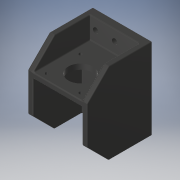
# Autodesk Inventor part: nema17_holder_z
Saved by Autodesk Inventor 2018 (Build 220112000, 112)
## iProperties
Created: 2018-06-01
Part Number: nema17_holder_z
Material: Plastic, Opaque Black
Document SubType Name: Modeling
Designer: Z. Deniz
Density: 0.952 g/cm^3
Appearance: Smooth - Black
Author: Z. Deniz
Autodesk Inventor part; units mm, degrees
ref_plane "YZ Plane" through (0, 0, 0) normal (1, 0, 0) x (0, 1, 0)
ref_plane "XZ Plane" through (0, 0, 0) normal (0, 1, 0) x (-1, 0, 0)
ref_plane "XY Plane" through (0, 0, 0) normal (0, 0, 1) x (1, 0, 0)
sketch "Sketch1" plane through (0, 0, 0) normal (0, 0, 1) x (1, 0, 0)
  line L0 (0, 0) -> (45, 0)
  line L1 (45, 0) -> (45, 75)
  line L2 (45, 75) -> (0, 75)
  line L3 (0, 75) -> (0, 0)
  line L4 (0, 55) -> (45, 55)
  line L5 (0, 50) -> (45, 50)
  line L6 (0, 75) -> (-5, 75)
  line L7 (-5, 75) -> (-5, 0)
  line L8 (-5, 0) -> (0, 0)
  line L9 (45, 75) -> (50, 75)
  line L10 (50, 75) -> (50, 0)
  line L11 (50, 0) -> (45, 0)
  dimension "d0" = 45
  dimension "d1" = 75
  dimension "d2" = 20
  dimension "d3" = 5
  dimension "d4" = 5
  dimension "d5" = 5
  constraints: 24 end point, 7 point on line, 6 perpendicular, 3 parallel, 1 horizontal
  measures "d0" distance of L2.end L1.end
  measures "d1" distance of L1.end L0.end
  measures "d2" distance between parallel lines of L4 L2
  measures "d3" distance between parallel lines of L5 L4
  measures "d4" distance of L2.end L6.end
  measures "d5" distance of L1.end L9.end
extrude "Extrusion1" add sketch "Sketch1" along normal blind 15 contours L3 L5 L1 L0 | L3 L2 L1 L4
extrude "Extrusion2" add sketch "Sketch1" along normal blind 60 contours L8 L7 L6 L3 | L1 L9 L10 L11 | L3 L4 L1 L5
chamfer "Chamfer1" distance 20 angle 45 4 edges at (47.5, 75, 60) (-2.5, 75, 60) (-2.5, 0, 60) (47.5, 0, 60)
sketch "Sketch2" plane through (0, 0, 15) normal (0, 0, 1) x (1, 0, 0)
  line L0 (0, 75) -> (0, 55) construction
  line L1 (0, 65) -> (45, 65) construction
  line L2 (45, 55) -> (45, 75) construction
  circle A0 centre (5, 65) radius 2.5
  circle A1 centre (22.5, 65) radius 2.5
  circle A2 centre (40, 65) radius 2.5
  line L3 (45, 55) -> (50, 55) projected
  line L4 (0, 75) -> (45, 75)
  line L5 (45, 75) -> (45, 55)
  line L6 (45, 55) -> (0, 55)
  line L7 (0, 55) -> (0, 75)
  point P0 (0, 0)
  dimension "d13" = 5
  dimension "d14" = 5
  dimension "d15" = 5
  dimension "d16" = 5
  dimension "d17" = 5
  dimension "d18" = 17.5
  constraints: 10 end point, 3 centre point, 3 midpoint, 2 parallel, 2 point on line, 1 horizontal, 1 perpendicular
  measures "d13" diameter of A0
  measures "d14" diameter of A1
  measures "d15" diameter of A2
  measures "d16" distance from line of L0 A0.centre
  measures "d17" distance from line of L2 A2.centre
  measures "d18" distance of A0.centre A1.centre
extrude "Extrusion3" cut sketch "Sketch2" against normal blind 15 contours A0 | A1 | A2
sketch "Sketch3" plane through (0, 55, 15) normal (0, 1, 0) x (1, 0, 0)
  line L0 (0, 0) -> (45, 0) construction
  line L1 (50, -45) -> (45, -45) construction
  line L2 (-5, -45) -> (0, -45) construction
  line L3 (45, 0) -> (45, -45) construction
  line L4 (7, -8.25) -> (38, -8.25) construction
  line L5 (38, -8.25) -> (38, -39.25) construction
  line L6 (38, -39.25) -> (7, -39.25) construction
  line L7 (7, -39.25) -> (7, -8.25) construction
  line L8 (7, -8.25) -> (38, -39.25) construction
  line L9 (38, -8.25) -> (7, -39.25) construction
  circle A0 centre (7, -8.25) radius 1.575
  circle A1 centre (38, -8.25) radius 1.575
  circle A2 centre (7, -39.25) radius 1.575
  circle A3 centre (38, -39.25) radius 1.575
  circle A4 centre (22.5, -23.75) radius 11.25
  line L10 (1.25, -2.5) -> (43.75, -2.5) construction
  line L11 (43.75, -2.5) -> (43.75, -45) construction
  line L12 (43.75, -45) -> (1.25, -45) construction
  line L13 (1.25, -45) -> (1.25, -2.5) construction
  line L14 (1.25, -2.5) -> (43.75, -45) construction
  line L15 (43.75, -2.5) -> (1.25, -45) construction
  line L16 (1.25, -2.5) -> (43.75, -45) construction
  line L17 (1.25, -45) -> (43.75, -2.5) construction
  line L18 (0, 0) -> (0, -25) projected
  point P0 (0, 15)
  dimension "d21" = 31
  dimension "d22" = 31
  dimension "d23" = 3.15
  dimension "d24" = 3.15
  dimension "d25" = 3.15
  dimension "d26" = 3.15
  dimension "d27" = 22.5
  dimension "d28" = 42.5
  dimension "d29" = 42.5
  dimension "d33" = 2.5
  dimension "d34" = 1.25
  constraints: 28 end point, 5 centre point, 5 coincident, 4 midpoint, 4 parallel, 2 horizontal, 2 perpendicular
  measures "d21" distance of L5.end L6.end
  measures "d22" distance of L4.end L5.end
  measures "d23" diameter of A0
  measures "d24" diameter of A1
  measures "d25" diameter of A2
  measures "d26" diameter of A3
  measures "d27" diameter of A4
  measures "d28" distance of L11.end L12.end
  measures "d29" distance of L10.end L11.end
  measures "d33" distance between parallel lines of L10 L0
  measures "d34" distance between parallel lines of L18 L13
extrude "Extrusion4" cut sketch "Sketch3" against normal blind 5
fillet "Fillet1" radius 1 42 edges at (-5, 37.5, 60) (-5, 10, 50) (0, 10, 50) (-2.5, 20, 60) (0, 35, 60) (22.5, 50, 60) (22.5, 55, 60) (-2.5, 55, 60) (-5, 65, 50) (0, 65, 50) (-2.5, 75, 40) (-5, 75, 20) (-5, 37.5, 0) (-2.5, 0, 40) (-5, 0, 20) (0, 0, 27.5) (22.5, 0, 15) (22.5, 0, 0) (0, 25, 15) (0, 50, 37.5) (22.5, 50, 15) (45, 35, 60) (50, 37.5, 60) (47.5, 20, 60) (50, 10, 50) (45, 10, 50) (47.5, 0, 40) (50, 0, 20) (45, 0, 27.5) (45, 25, 15) (45, 50, 37.5) (50, 65, 50) (47.5, 55, 60) (47.5, 75, 40) (45, 65, 50) (45, 75, 27.5) (50, 75, 20) (22.5, 75, 0) (45, 55, 37.5) (0, 55, 37.5) (50, 37.5, 0) (0, 75, 27.5)
extrude "Extrusion5" cut sketch "Sketch2" against normal blind 7.5
fillet "Fillet2" radius 1 8 edges at (0, 65, 7.5) (0, 75, 11.25) (0, 55, 11.25) (22.5, 55, 7.5) (22.5, 75, 7.5) (45, 75, 11.25) (45, 55, 11.25) (45, 65, 7.5)
body "Solid1"
